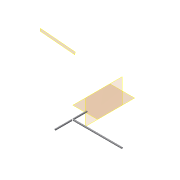
# Autodesk Inventor part: 00_Beampath_Coupling
Saved by Autodesk Inventor 2019.4 (Build 234330000, 330)
## iProperties
Created: 2021-01-13
Part Number: 00_Beampath_Coupling
Material: Generic
Document SubType Name: Modeling
Designer: diederichbenedict
Density: 1 g/cm^3
Appearance: Default
Author: diederichbenedict
Autodesk Inventor part; units mm, degrees
ref_plane "YZ Plane" through (0, 0, 0) normal (1, 0, 0) x (0, 1, 0)
ref_plane "XZ Plane" through (0, 0, 0) normal (0, 1, 0) x (-1, 0, 0)
ref_plane "XY Plane" through (0, 0, 0) normal (0, 0, 1) x (1, 0, 0)
ref_plane "Work Plane1" through (188.6118, -245.1178, 0) normal (0, 0, 1) x (-0.9961, 0.0884, 0)
sketch "Sketch1" plane through (188.6118, -245.1178, 0) normal (0, 0, 1) x (-0.9961, 0.0884, 0)
  circle A0 centre (0, 0) radius 2.6486 projected
  circle A1 centre (0, 0) radius 1
  point P0 (209.5331, -227.4929)
  dimension "d0" = 2
  constraints: 1 centre point, 1 coincident
  measures "d0" diameter of A1
extrude "Extrusion1" add sketch "Sketch1" along normal blind 45 contours A1
ref_plane "Work Plane2" through (188.6118, -261.1178, -48) normal (1, 0, 0) x (0, 1, 0)
sketch "Sketch2" plane through (188.6118, -261.1178, -48) normal (1, 0, 0) x (0, 1, 0)
  line L0 (17, 93) -> (15, 93) projected
  line L1 (15, 48) -> (17, 48) projected
  circle A0 centre (16, 68) radius 1
  line L2 (15, 48) -> (15, 93) projected
  point P0 (261.1178, 48)
  dimension "d8" = 20
  constraints: 1 centre point, 1 tangent
  measures "d8" distance from line of A0.centre L1
extrude "Extrusion2" add sketch "Sketch2" along normal blind 70
ref_plane "Work Plane3" through (172.6118, -245.1178, 98) normal (0, 1, 0) x (1, 0, 0)
sketch "Sketch3" plane through (172.6118, -245.1178, 98) normal (0, 1, 0) x (1, 0, 0)
  line L0 (86, 77) -> (86, 79) projected
  line L1 (15, 53) -> (17, 53) projected
  line L2 (17, 98) -> (15, 98) projected
  line L3 (17, 77) -> (5.6178, 88.3822)
  line L4 (5.6178, 88.3822) -> (4.9785, 87.7429)
  line L5 (4.9785, 87.7429) -> (17, 75.7215)
  line L6 (17, 75.7215) -> (17, 77)
  line L7 (17, 98) -> (17, 53) projected
  point P0 (-172.6118, 98)
  point P1 (16, 68)
  point P2 (16, 68)
  point P3 (16, 68)
  point P4 (16, 68)
  constraints: 8 end point, 3 point on line, 2 perpendicular, 2 other
extrude "Extrusion3" cut sketch "Sketch3" along normal mid plane 50
body "Solid1"
